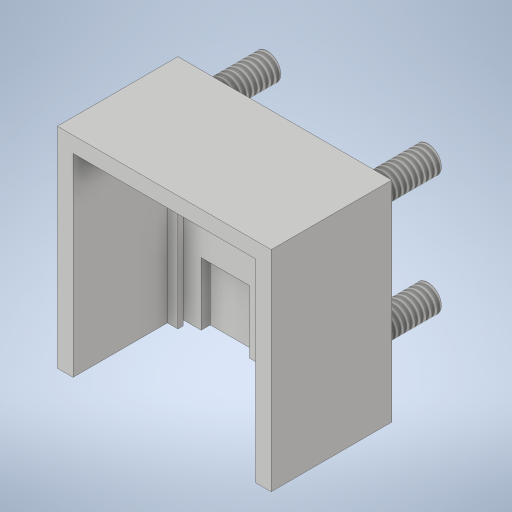
# Autodesk Inventor part: ecog_casing_1
Saved by Autodesk Inventor 2023 (Build 270158000, 158)
## iProperties
Created: 2020-02-18
Part Number: ecog_casing_1
Material: Generic
Document SubType Name: Modeling
Designer: bgereke
Density: 1 g/cm^3
Appearance: Default
Author: bgereke
Autodesk Inventor part; units mm, degrees
ref_plane "YZ Plane" through (0, 0, 0) normal (1, 0, 0) x (0, 1, 0)
ref_plane "XZ Plane" through (0, 0, 0) normal (0, 1, 0) x (-1, 0, 0)
ref_plane "XY Plane" through (0, 0, 0) normal (0, 0, 1) x (1, 0, 0)
sketch "Sketch1" plane through (0, 0, 0) normal (0, 0, 1) x (1, 0, 0)
  line L0 (0, 0) -> (38, 0)
  line L1 (38, 0) -> (38, 40)
  line L2 (38, 40) -> (0, 40)
  line L3 (0, 40) -> (0, 0)
  dimension "d0" = 38
  dimension "d1" = 40
  constraints: 8 end point, 2 parallel, 1 horizontal, 1 perpendicular
  measures "d0" distance of L2.end L1.end
  measures "d1" distance of L1.end L0.end
extrude "Extrusion1" add sketch "Sketch1" along normal blind 3
sketch "Sketch2" plane through (0, 0, 3) normal (0, 0, 1) x (1, 0, 0)
  line L0 (38, 0) -> (38, 40) projected
  line L1 (38, 40) -> (38, 0)
  line L2 (38, 0) -> (34.9318, 0)
  line L3 (35, 37) -> (3, 37)
  line L4 (3, 37) -> (3, 0)
  line L5 (0, 40) -> (0, 0) projected
  line L6 (0, 0) -> (0, 40)
  line L7 (38, 40) -> (0, 40) projected
  line L8 (0, 40) -> (38, 40)
  line L9 (35, 37) -> (35, 0)
  line L10 (3, 0) -> (0, 0)
  dimension "d4" = 3
  dimension "d5" = 3
  dimension "d6" = 3
  constraints: 16 end point, 2 collinear, 2 horizontal, 1 perpendicular, 1 point on line
  measures "d4" distance between parallel lines of L0 L9
  measures "d5" distance between parallel lines of L7 L3
  measures "d6" distance between parallel lines of L5 L4
extrude "Extrusion2" add sketch "Sketch2" along normal blind 20
sketch "Sketch3" plane through (38, 0, 0) normal (1, 0, 0) x (0, 0, -1)
  line L0 (-23, 0) -> (-23, 40) projected
  line L1 (0, 0) -> (-23, 0)
  line L2 (-23, 0) -> (-23, 40)
  line L3 (-23, 40) -> (0, 40)
  line L4 (0, 40) -> (0, 0)
  constraints: 8 end point, 2 parallel, 1 horizontal, 1 perpendicular
extrude "Extrusion3" add sketch "Sketch3" along normal blind 1.4
sketch "Sketch4" plane through (35, 0, 3) normal (-1, 0, 0) x (0, 0, 1)
  line L0 (0, 37) -> (20, 37) projected
  line L1 (0, 0) -> (20, 0) projected
  line L2 (20, 37) -> (0, 37)
  line L3 (0, 37) -> (0, 0)
  line L4 (0, 0) -> (20, 0)
  line L5 (20, 0) -> (20, 37)
  point P0 (-3, 0)
  constraints: 8 end point, 2 parallel, 1 horizontal, 1 perpendicular
extrude "Extrusion4" cut sketch "Sketch4" against normal blind 1.4
sketch "Sketch5" plane through (0, 0, 0) normal (-1, 0, 0) x (0, 0, 1)
  line L0 (0, 40) -> (23, 40) projected
  line L1 (23, 40) -> (0, 40)
  line L2 (0, 40) -> (0, 0)
  line L3 (0, 0) -> (23, 0)
  line L4 (23, 0) -> (23, 40)
  constraints: 8 end point, 2 parallel, 1 horizontal, 1 perpendicular
extrude "Extrusion5" add sketch "Sketch5" along normal blind 1.4
sketch "Sketch6" plane through (3, 0, 3) normal (1, 0, 0) x (0, 0, -1)
  line L0 (0, 37) -> (0, 0) projected
  line L1 (-20, 0) -> (-20, 37) projected
  line L2 (0, 37) -> (-20, 37)
  line L3 (-20, 37) -> (-20, 0)
  line L4 (-20, 0) -> (0, 0)
  line L5 (0, 0) -> (0, 37)
  point P0 (3, 0)
  constraints: 8 end point, 2 parallel, 1 horizontal, 1 perpendicular
extrude "Extrusion6" cut sketch "Sketch6" against normal blind 1.4
sketch "Sketch7" plane through (39.4, 0, 0) normal (0, -1, 0) x (1, 0, 0)
  line L0 (-3, 3) -> (-3, 23) projected
  line L1 (-3, 4) -> (-5, 4)
  line L2 (-5, 4) -> (-5, 5)
  line L3 (-5, 5) -> (-3, 5)
  line L4 (-3, 5) -> (-3, 4)
  line L5 (-37.8, 3) -> (-3, 3) projected
  point P0 (-39.4, 0)
  dimension "d17" = 2
  dimension "d18" = 1
  dimension "d19" = 1
  constraints: 8 end point, 2 parallel, 1 horizontal, 1 perpendicular, 1 point on line
  measures "d17" distance of L2.end L3.end
  measures "d18" distance of L1.end L2.end
  measures "d19" distance between parallel lines of L5 L1
extrude "Extrusion7" add sketch "Sketch7" against normal blind 37.0078
sketch "Sketch9" plane through (39.4, 0, 0) normal (0, -1, 0) x (1, 0, 0)
  line L0 (-37.8, 3) -> (-37.8, 23) projected
  line L1 (-37.8, 4) -> (-35.8, 4)
  line L2 (-35.8, 4) -> (-35.8, 5)
  line L3 (-35.8, 5) -> (-37.8, 5)
  line L4 (-37.8, 5) -> (-37.8, 4)
  line L5 (-37.8, 3) -> (-3, 3) projected
  point P0 (-39.4, 0)
  dimension "d22" = 2
  dimension "d23" = 1
  dimension "d24" = 1
  constraints: 8 end point, 2 parallel, 1 horizontal, 1 perpendicular, 1 point on line
  measures "d22" distance of L3.end L2.end
  measures "d23" distance of L2.end L1.end
  measures "d24" distance between parallel lines of L5 L1
extrude "Extrusion8" add sketch "Sketch9" against normal blind 37.0078
sketch "Sketch10" plane through (1.6, 37, 3) normal (0, -1, 0) x (1, 0, 0)
  line L0 (0, 2) -> (2, 2) projected
  line L1 (32.8, 1) -> (32.8, 2) projected
  line L2 (2, 2) -> (32.8, 2)
  line L3 (32.8, 2) -> (32.8, 1)
  line L4 (32.8, 1) -> (2, 1)
  line L5 (2, 1) -> (2, 2)
  point P0 (-1.6, -3)
  constraints: 8 end point, 2 parallel, 1 horizontal, 1 perpendicular
extrude "Extrusion9" add sketch "Sketch10" along normal blind 2
sketch "Sketch11" plane through (1.6, 0, 3) normal (1, 0, 0) x (0, 0, -1)
  line L0 (-1, 37) -> (0, 37) projected
  line L1 (0, 0) -> (-1, 0) projected
  line L2 (0, 37) -> (-1, 37)
  line L3 (-1, 37) -> (-1, 0)
  line L4 (-1, 0) -> (0, 0)
  line L5 (0, 0) -> (0, 37)
  point P0 (3, 0)
  constraints: 8 end point, 2 parallel, 1 horizontal, 1 perpendicular
extrude "Extrusion10" add sketch "Sketch11" along normal blind 1
sketch "Sketch12" plane through (36.4, 0, 3) normal (-1, 0, 0) x (0, 0, 1)
  line L0 (0, 0) -> (0, 37) projected
  line L1 (1, 0) -> (0, 0) projected
  line L2 (0, 37) -> (1, 37)
  line L3 (1, 37) -> (1, 0)
  line L4 (1, 0) -> (0, 0)
  line L5 (0, 0) -> (0, 37)
  point P0 (-3, 0)
  constraints: 8 end point, 2 parallel, 1 horizontal, 1 perpendicular
extrude "Extrusion11" add sketch "Sketch12" along normal blind 1
sketch "Sketch13" plane through (39.4, 0, 0) normal (0, -1, 0) x (1, 0, 0)
  line L0 (-4, 3) -> (-36.8, 3) projected
  line L1 (-33.371, 3) -> (-24.171, 3)
  line L2 (-24.171, 3) -> (-24.171, 1.25)
  line L3 (-24.171, 1.25) -> (-33.371, 1.25)
  line L4 (-33.371, 1.25) -> (-33.371, 3)
  line L5 (-16.671, 3) -> (-7.471, 3)
  line L6 (-7.471, 3) -> (-7.471, 1.25)
  line L7 (-7.471, 1.25) -> (-16.671, 1.25)
  line L8 (-16.671, 1.25) -> (-16.671, 3)
  point P0 (-39.4, 0)
  dimension "d33" = 9.2
  dimension "d34" = 9.2
  dimension "d35" = 7.5
  dimension "d36" = 3.429
  dimension "d37" = 1.75
  constraints: 16 end point, 4 parallel, 3 point on line, 2 horizontal, 2 perpendicular
  measures "d33" distance between parallel lines of L4 L2
  measures "d34" distance between parallel lines of L6 L8
  measures "d35" distance between parallel lines of L2 L8
  measures "d36" distance of L0.end L1.start
  measures "d37" distance of L1.end L2.end
extrude "Extrusion12" cut sketch "Sketch13" against normal blind 12
sketch "Sketch14" plane through (0, 0, 0) normal (0, 0, -1) x (-1, 0, 0)
  circle A0 centre (-3.68, 12) radius 2.54
  circle A1 centre (-19, 23.43) radius 2.54
  circle A2 centre (-3.68, 34.92) radius 2.54
  circle A3 centre (-34.32, 12) radius 2.54
  circle A4 centre (-34.32, 34.92) radius 2.54
  line L0 (1.4, 0) -> (-39.4, 0) projected
  line L1 (1.4, 40) -> (1.4, 0) projected
  line L2 (-39.4, 0) -> (-39.4, 40) projected
  line L3 (1.4, 40) -> (-39.4, 40) projected
  point P0 (0, 0)
  dimension "d40" = 5.08
  dimension "d41" = 5.08
  dimension "d42" = 5.08
  dimension "d43" = 5.08
  dimension "d44" = 5.08
  dimension "d45" = 12
  dimension "d46" = 12
  dimension "d47" = 5.08
  dimension "d48" = 5.08
  dimension "d49" = 5.08
  dimension "d50" = 5.08
  dimension "d51" = 5.08
  dimension "d52" = 5.08
  dimension "d53" = 11.43
  constraints: 5 centre point
  measures "d40" diameter of A0
  measures "d41" diameter of A1
  measures "d42" diameter of A2
  measures "d43" diameter of A3
  measures "d44" diameter of A4
  measures "d45" distance from line of L0 A0.centre
  measures "d46" distance from line of L0 A3.centre
  measures "d47" distance from line of L1 A0.centre
  measures "d48" distance from line of L2 A3.centre
  measures "d49" distance from line of L1 A2.centre
  measures "d50" distance from line of L3 A2.centre
  measures "d51" distance from line of L2 A4.centre
  measures "d52" distance from line of L3 A4.centre
  measures "d53" vertical distance of A3.centre A1.centre
extrude "Extrusion13" add sketch "Sketch14" along normal blind 12 contours A0 | A1 | A2 | A3 | A4
thread "Thread1" size "12-24 UNC" class "2A" standard "ANSI Unified Screw Threads" full length
thread "Thread2" size "12-24 UNC" class "2A" standard "ANSI Unified Screw Threads" full length
thread "Thread3" size "12-24 UNC" class "2A" standard "ANSI Unified Screw Threads" full length
thread "Thread4" size "12-24 UNC" class "2A" standard "ANSI Unified Screw Threads" full length
thread "Thread5" size "12-24 UNC" class "2A" standard "ANSI Unified Screw Threads" full length
body "Solid1"
